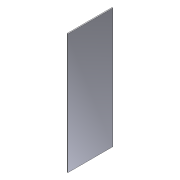
# Autodesk Inventor part: VerticalJagTower
Saved by Autodesk Inventor 2012 (Build 160160000, 160)
## iProperties
Created: 2012-01-22
Part Number: VerticalJagTower
Material: ABS Plastic
Document SubType Name: Modeling
Designer: JesseK
Density: 1.06 g/cm^3
Mass: 208.443 g
Surface Area: 1274.19 cm^2
Volume: 196.645 cm^3
Author: JesseK
Autodesk Inventor part; units mm, degrees
ref_plane "YZ Plane" through (0, 0, 0) normal (1, 0, 0) x (0, 1, 0)
ref_plane "XZ Plane" through (0, 0, 0) normal (0, 1, 0) x (-1, 0, 0)
ref_plane "XY Plane" through (0, 0, 0) normal (0, 0, 1) x (1, 0, 0)
sketch "Sketch1" plane through (0, 0, 0) normal (0, 0, 1) x (1, 0, 0)
  line L0 (0, 0) -> (3.175, 0)
  line L1 (3.175, 0) -> (3.175, 406.4)
  line L2 (3.175, 406.4) -> (0, 406.4)
  line L3 (0, 406.4) -> (0, 0)
  dimension "d0" = 3.175
  dimension "d1" = 406.4
  constraints: 8 end point, 2 parallel, 1 horizontal, 1 perpendicular
  measures "d0" distance of L1.end L2.end
  measures "d1" distance of L0.end L1.end
extrude "Extrusion1" add sketch "Sketch1" along normal blind 152.4
body "Solid1"
